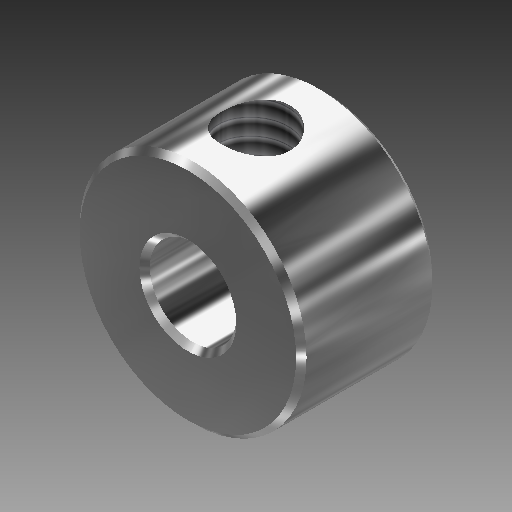
# Autodesk Inventor part: Shaft Collar
Saved by Autodesk Inventor 2018 (Build 220112000, 112)
## iProperties
Created: 2010-06-21
Part Number: Shaft Collar
Document SubType Name: Modeling
Designer: Phil
Density: 1 g/cm^3
Material: Generic
Appearance: Chrome - Polished
Author: Phil
Autodesk Inventor part; units mm, degrees
note: some values were not read from the file. Chosen so that the rebuilt part matches the saved one: direction of "Hole2".
ref_plane "YZ Plane" through (0, 0, 0) normal (1, 0, 0) x (0, 1, 0)
ref_plane "XY Plane" through (0, 0, 0) normal (0, 0, 1) x (1, 0, 0)
sketch "Sketch1" plane through (0, 0, 0) normal (0, 0, 1) x (1, 0, 0)
  circle A0 centre (0, 0) radius 5.4991
  dimension "d0" = 10.9982
  constraints: 1 centre point, 1 coincident
  measures "d0" diameter of A0
extrude "Extrusion1" add sketch "Sketch1" against normal blind 6.604
chamfer "Chamfer1" distance 0.254 angle 45 2 edges at (-5.4991, 0, 0) (-5.4991, 0, -6.604)
sketch "Sketch2" plane through (0, 0, 0) normal (0, 0, 1) x (1, 0, 0)
  circle A0 centre (0, 0) radius 5.2451 projected
hole "Hole1" at (0, 0, 0) direction (0, 0, -1) diameter 4.191 end through all
ref_plane "Work Plane1" through (0, 5.4991, 0) normal (0, 1, 0) x (-1, 0, 0)
sketch "Sketch3" plane through (0, 5.4991, 0) normal (0, 1, 0) x (-1, 0, 0)
  line L0 (-5.2451, 0) -> (5.2451, 0) projected
  line L1 (5.4991, -0.254) -> (5.4991, -6.35) projected
  point P0 (0, 0)
  point P1 (0, -3.302)
hole "Hole2" at (0, 5.4991, -3.302) direction (0, -1, 0) diameter 3.302 end up to surface thread size "8-32 UNC" class "2B" standard "ANSI Unified Screw Threads"
chamfer "Chamfer2" distance 0.254 angle 45 2 edges at (0, 2.0955, 0) (0, 2.0955, -6.604)
body "Solid1"
